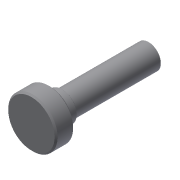
# Autodesk Inventor part: Shoulder Screw
Saved by Autodesk Inventor 2017 (Build 210142000, 142)
## iProperties
Created: 2016-07-28
Part Number: Shoulder Screw
Material: Generic
Document SubType Name: Modeling
Designer: Tutorial Books
Density: 1 g/cm^3
Appearance: Default
Author: Tutorial Books
Autodesk Inventor part; units mm, degrees
ref_plane "YZ Plane" through (0, 0, 0) normal (1, 0, 0) x (0, 1, 0)
ref_plane "XZ Plane" through (0, 0, 0) normal (0, 1, 0) x (-1, 0, 0)
ref_plane "XY Plane" through (0, 0, 0) normal (0, 0, 1) x (1, 0, 0)
sketch "Sketch1" plane through (0, 0, 0) normal (1, 0, 0) x (0, 1, 0)
  line L0 (25.4, 0) -> (25.4, 19.05)
  line L1 (25.4, 19.05) -> (0, 19.05)
  line L2 (0, 19.05) -> (0, -101.6)
  line L3 (0, -101.6) -> (12.7, -101.6)
  line L4 (12.7, -101.6) -> (12.7, -12.7)
  line L5 (12.7, -12.7) -> (15.24, -12.7)
  line L6 (15.24, -12.7) -> (15.24, 0)
  line L7 (15.24, 0) -> (25.4, 0)
  point P0 (0, 0)
  dimension "d10" = 0.508
  dimension "d0" = 19.05
  dimension "d1" = 25.4
  dimension "d2" = 12.7
  dimension "d3" = 15.24
  dimension "d4" = 120.65
  dimension "d5" = 88.9
  constraints: 16 end point, 7 perpendicular, 2 point on line, 1 vertical
  measures "d0" distance of L0.start L0.end
  measures "d1" distance of L0.end L1.end
  measures "d2" distance of L2.end L3.end
  measures "d3" distance between parallel lines of L2 L6
  measures "d4" distance between parallel lines of L3 L1
  measures "d5" distance between parallel lines of L3 L5
revolve "Revolution1" add sketch "Sketch1" angle 360 about axis through (0, 0, 19.05) along (0, 0, -1)
chamfer "Chamfer1" distance 1.524 angle 45 2 edges at (0, -25.4, 19.05) (0, -25.4, 0)
fillet "Fillet1" radius 0.508 3 edges at (0, -15.24, 0) (0, -15.24, -12.7) (0, -12.7, -12.7)
body "Solid1"
